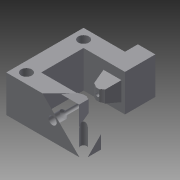
# Autodesk Inventor part: OfflineBowdenExtruder
Saved by Autodesk Inventor 2015 SP1 (Build 190203100, 203)
## iProperties
Created: 2015-04-29
Part Number: OfflineBowdenExtruder
Material: Generic
Document SubType Name: Modeling
Designer: Jack
Density: 1 g/cm^3
Appearance: Default
Author: Jack
Autodesk Inventor part; units mm, degrees
ref_plane "YZ Plane" through (0, 0, 0) normal (1, 0, 0) x (0, 1, 0)
ref_plane "XZ Plane" through (0, 0, 0) normal (0, 1, 0) x (-1, 0, 0)
ref_plane "XY Plane" through (0, 0, 0) normal (0, 0, 1) x (1, 0, 0)
sketch "Sketch1" plane through (0, 0, 0) normal (0, 0, 1) x (1, 0, 0)
  line L0 (0, 0) -> (42, 0)
  line L1 (0, 0) -> (0, 42)
  line L2 (32, 32.5) -> (9.5, 32.5)
  line L3 (9.5, 32.5) -> (9.5, 9.5)
  line L4 (9.5, 9.5) -> (42, 9.5)
  line L5 (42, 9.5) -> (42, 0)
  line L6 (0, 42) -> (20, 42)
  line L7 (20, 42) -> (20, 49)
  line L8 (20, 49) -> (32, 49)
  line L9 (32, 49) -> (32, 32.5)
  dimension "d0" = 42
  dimension "d1" = 42
  dimension "d5" = 9.5
  dimension "d6" = 9.5
  dimension "d21" = 32
  dimension "d22" = 7
  dimension "d23" = 9.5
  dimension "d24" = 12
  constraints: 20 end point, 5 perpendicular, 3 vertical, 2 horizontal
  measures "d0" distance of L0.start L0.end
  measures "d1" distance of L0.start L1.end
  measures "d5" distance between parallel lines of L0 L4
  measures "d6" distance between parallel lines of L1 L3
  measures "d21" distance between parallel lines of L9 L1
  measures "d22" distance of L6.end L7.end
  measures "d23" distance between parallel lines of L6 L2
  measures "d24" distance between parallel lines of L9 L7
extrude "Extrusion1" add sketch "Sketch1" along normal blind 20
sketch "Sketch2" plane through (0, 0, 20) normal (0, 0, 1) x (1, 0, 0)
  line L0 (0, 42) -> (0, 0) projected
  line L1 (20, 42) -> (0, 42) projected
  point P0 (5.5, 36.5)
  point P1 (5.5, 5.5)
  dimension "d9" = 31
  dimension "d13" = 5.5
  dimension "d25" = 5.5
  constraints: 1 vertical alignment
  measures "d9" distance of point (5.5, 5.5) point (5.5, 36.5)
  measures "d13" distance from line of L0 point (5.5, 5.5)
  measures "d25" distance from line of L1 point (5.5, 36.5)
hole "Hole1" at (5.5, 36.5, 20) at (5.5, 5.5, 20) direction (0, 0, -1) diameter 3.5 end through all counterbore diameter 5.8 counterbore depth 14
sketch "Sketch3" plane through (0, 0, 20) normal (0, 0, 1) x (1, 0, 0)
  circle A0 centre (5.5, 5.5) radius 2.9 projected
  point P0 (36.5, 5.5)
  dimension "d26" = 31
  constraints: 1 horizontal alignment
  measures "d26" distance of A0.centre point (36.5, 5.5)
hole "Hole2" at (36.5, 5.5, 20) direction (0, 0, -1) diameter 3.5 end through all counterbore diameter 5.8 counterbore depth 3.5
sketch "Sketch4" plane through (9.5, 32.5, 0) normal (0, -1, 0) x (1, 0, 0)
  line L0 (22.5, 0) -> (22.5, 20) projected
  line L1 (0, 20) -> (22.5, 20) projected
  line L2 (12.7, 7) -> (18.7, 7)
  line L3 (18.7, 7) -> (18.7, 13)
  line L4 (18.7, 13) -> (12.7, 13)
  line L5 (12.7, 13) -> (12.7, 7)
  point P0 (-9.5, 0)
  dimension "d34" = 6
  dimension "d35" = 6
  dimension "d36" = 7
  dimension "d37" = 3.8
  constraints: 8 end point, 2 parallel, 1 horizontal, 1 perpendicular
  measures "d34" distance of L3.end L4.end
  measures "d35" distance of L2.end L3.end
  measures "d36" distance between parallel lines of L1 L4
  measures "d37" distance between parallel lines of L0 L3
extrude "Extrusion2" add sketch "Sketch4" along normal blind 7
sketch "Sketch5" plane through (9.5, 9.5, 0) normal (0, 1, 0) x (1, 0, 0)
  line L0 (12.7, -7) -> (18.7, -7) projected
  line L1 (18.7, -7) -> (18.7, -13) projected
  line L2 (18.7, -13) -> (12.7, -13) projected
  line L3 (12.7, -13) -> (12.7, -7) projected
  point P0 (-9.5, 0)
extrude "Extrusion3" add sketch "Sketch5" along normal blind 7
sketch "Sketch8" plane through (22.2, 9.5, 13) normal (0, 0, 1) x (1, 0, 0)
  line L0 (0, 7) -> (6, 7) projected
  line L1 (0, 0) -> (0, 7) projected
  line L2 (6, 7) -> (0, 7) projected
  line L3 (2, 7) -> (2, 9) construction
  line L4 (4, 7) -> (4, 9) construction
  arc A0 (0, 7) -> (2, 8.1162) centre (-1.2, 11.5) ccw
  arc A1 (4, 8.1162) -> (6, 7) centre (7.2, 11.5) ccw
  line L5 (2, 8.1162) -> (4, 8.1162)
  point P0 (-22.2, -9.5)
  dimension "d58" = 2
  dimension "d59" = 2
  dimension "d60" = 2
  dimension "d61" = 1.2
  dimension "d62" = 4.5
  constraints: 6 end point, 4 point on circle, 4 point on line, 2 centre point, 2 horizontal alignment, 2 vertical, 1 horizontal
  measures "d58" distance between parallel lines of L4 L3
  measures "d59" distance between parallel lines of L1 L3
  measures "d60" distance of L4.start L4.end
  measures "d61" distance from line of L1 A0.centre
  measures "d62" distance from line of L0 A0.centre
extrude "Extrusion5" add sketch "Sketch8" against normal up to surface (6 mm away)
sketch "Sketch9" plane through (22.2, 32.5, 13) normal (0, 0, 1) x (1, 0, 0)
  line L0 (0, 0) -> (0, -7) projected
  line L1 (6, -7) -> (0, -7) projected
  line L2 (6, 0) -> (6, -7) projected
  arc A0 (2, -8.1162) -> (0, -7) centre (-1.2, -11.5) ccw
  line L3 (2, -7) -> (2, -9) construction
  line L4 (4, -7) -> (4, -9) construction
  arc A1 (6, -7) -> (4, -8.1162) centre (7.2, -11.5) ccw
  line L5 (2, -8.1162) -> (4, -8.1162)
  point P0 (-22.2, -32.5)
  dimension "d66" = 1.2
  dimension "d67" = 4.5
  dimension "d68" = 2
  dimension "d69" = 2
  dimension "d70" = 2
  constraints: 6 end point, 4 point on circle, 4 point on line, 2 centre point, 2 horizontal alignment, 2 vertical, 1 horizontal
  measures "d66" distance from line of L0 A0.centre
  measures "d67" distance from line of A0.centre L1
  measures "d68" distance of L4.start L4.end
  measures "d69" distance between parallel lines of L2 L4
  measures "d70" distance between parallel lines of L4 L3
extrude "Extrusion6" add sketch "Sketch9" against normal up to surface (6 mm away)
sketch "Sketch10" plane through (0, 0, 0) normal (0, -1, 0) x (1, 0, 0)
  line L0 (28.2, 13) -> (22.2, 13) projected
  line L1 (28.2, 13) -> (26.2, 13) projected
  line L2 (26.2, 13) -> (24.2, 13) projected
  line L3 (24.2, 13) -> (22.2, 13) projected
  line L4 (22.2, 7) -> (28.2, 7) projected
  line L5 (28.2, 7) -> (28.2, 13) projected
  line L6 (22.2, 13) -> (22.2, 7) projected
  point P0 (25.2, 10)
  dimension "d82" = 3
  dimension "d83" = 3
  measures "d82" distance from line of L5 point (25.2, 10)
  measures "d83" distance from line of L0 point (25.2, 10)
hole "Hole4" at (25.2, 0, 10) direction (0, 1, 0) diameter 2 end through all counterbore diameter 4.4 counterbore depth 6
draft "FaceDraft1" angle 15 pull direction (0, -1, 0) faces at (22.2, 30.1667, 11) fixed edges at (22.2, 25.5, 10)
draft "FaceDraft2" angle 15 pull direction (0, -1, 0) faces at (23.8166, 30.0802, 13) fixed edges at (25.2, 24.3838, 13)
draft "FaceDraft3" angle 15 pull direction (0, -1, 0) faces at (28.2, 30.1667, 11.8246) fixed edges at (28.2, 25.5, 10.1495)
draft "FaceDraft4" angle 15 pull direction (0, -1, 0) faces at (25.9582, 30.0802, 7) fixed edges at (25.2, 24.3838, 7)
draft "FaceDraft5" angle 15 pull direction (0, 1, 0) faces at (24.4418, 11.9198, 13) fixed edges at (25.2, 17.6162, 13)
draft "FaceDraft6" angle 15 pull direction (0, 1, 0) faces at (28.2, 11.8333, 11.8246) fixed edges at (28.2, 16.5, 10.1495)
draft "FaceDraft7" angle 15 pull direction (0, 1, 0) faces at (26.5834, 11.9198, 7) fixed edges at (25.2, 17.6162, 7)
draft "FaceDraft8" angle 15 pull direction (0, 1, 0) faces at (22.2, 11.8333, 8.9003) fixed edges at (22.2, 16.5, 10)
chamfer "Chamfer1" distance 1.2 angle 45 1 edges at (25.2, 6, 11)
sketch "Sketch11" plane through (20, 49, 0) normal (0, 1, 0) x (1, 0, 0)
  circle A0 centre (5.2, -10) radius 1 projected
  point P0 (-20, 0)
hole "Hole5" at (25.2, 49, 10) direction (0, -1, 0) diameter 2 end through all counterbore diameter 9.4 counterbore depth 11
body "Solid1"
